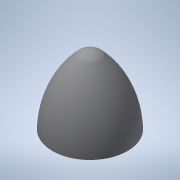
# Autodesk Inventor part: 風扇頭
Saved by Autodesk Inventor 2020 (Build 240168000, 168)
## iProperties
Created: 2017-11-27
Part Number: 風扇頭
Material: 一般
Document SubType Name: Modeling
Designer: USER
Density: 1 g/cm^3
Appearance: Default
Author: USER
Autodesk Inventor part; units mm, degrees
ref_plane "YZ Plane" through (0, 0, 0) normal (1, 0, 0) x (0, 1, 0)
ref_plane "XZ Plane" through (0, 0, 0) normal (0, 1, 0) x (-1, 0, 0)
sketch "草圖1" plane through (0, 0, 0) normal (0, 0, 1) x (1, 0, 0)
  circle A0 centre (0, 0) radius 10.85
  dimension "d0" = 21.7
  constraints: 1 centre point, 1 coincident
  measures "d0" diameter of A0
extrude "擠出1" add sketch "草圖1" along normal blind 18.7
sketch "草圖2" plane through (0, 0, 0) normal (1, 0, 0) x (0, 1, 0)
  line L0 (-2.85, 22.2303) -> (-2.85, 15.6814) construction
  line L1 (2.85, 22.4738) -> (2.85, 15.3185) construction
  line L2 (0, 0) -> (0, 5.3746) construction
  line L3 (-10.85, 0) -> (10.85, 0) projected
  line L4 (10.85, 18.7) -> (-10.85, 18.7) projected
  arc A0 (-2.85, 18.7) -> (-10.85, 0) centre (16.1456, -0.4877) ccw
  arc A1 (10.85, 0) -> (2.85, 18.7) centre (-16.1456, -0.4877) ccw construction
  line L5 (-10.85, 0) -> (-10.85, 18.7) projected
  line L6 (-2.85, 18.7) -> (-10.85, 18.7)
  line L7 (0, -5.08) -> (0, 27.0661) projected
  dimension "d3" = 5.7
  dimension "d4" = 2.85
  dimension "d6" = 27
  constraints: 8 end point, 4 point on circle, 3 vertical, 2 centre point, 2 point on line, 2 symmetric about line, 1 perpendicular, 1 other
  measures "d3" distance between parallel lines of L1 L0
  measures "d4" distance between parallel lines of L2 L1
  measures "d6" radius of A0
revolve "迴轉1" cut sketch "草圖2" angle 360 about axis through (0, 0, -10) along (0, 0, 1) contours L5 L4 A0
sketch "草圖3" plane through (0, 0, 0) normal (0, 1, 0) x (-1, 0, 0)
  line L0 (2.85, 18.7) -> (-2.85, 18.7) projected
  line L1 (0, 18.7) -> (0, 19.7)
  arc A0 (2.85, 18.7) -> (0, 19.7) centre (0.0215, 15.2001) ccw
  line L2 (0, 18.7) -> (2.85, 18.7)
  line L3 (0, -3.9893) -> (0, 23.9355) projected
  point P0 (0, 0)
  dimension "d10" = 1
  dimension "d11" = 4.5
  constraints: 4 end point, 2 point on circle, 1 centre point, 1 collinear, 1 midpoint, 1 vertical
  measures "d10" distance from line of L1.end L0
  measures "d11" radius of A0
revolve "迴轉2" add sketch "草圖3" angle 360 about axis through (0, 0, -10) along (0, 0, 1)
ref_plane "工作平面1" through (0, 0, 18.7) normal (0, 0, -1) x (-1, 0, 0)
sketch "草圖4" plane through (0, 0, 18.7) normal (0, 0, -1) x (-1, 0, 0)
  line L0 (0, -1.1547) -> (-1, -0.5774)
  line L1 (-1, -0.5774) -> (-1, 0.5774)
  line L2 (-1, 0.5774) -> (0, 1.1547)
  line L3 (0, 1.1547) -> (1, 0.5774)
  line L4 (1, 0.5774) -> (1, -0.5774)
  line L5 (1, -0.5774) -> (0, -1.1547)
  line L6 (0, 0) -> (0, 2.3379) construction
  dimension "d14" = 2
  constraints: 14 end point, 1 coincident, 1 parallel, 1 vertical, 13 other
  measures "d14" distance between parallel lines of L1 L4
